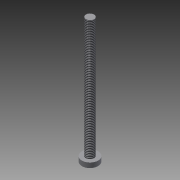
# Autodesk Inventor part: 6-32_Bolt
Saved by Autodesk Inventor 2015 (Build 190159000, 159)
## iProperties
Created: 2017-03-10
Part Number: 6-32_Bolt
Material: Generic
Document SubType Name: Modeling
Designer: Ernest
Density: 1 g/cm^3
Appearance: Default
Author: Ernest
Autodesk Inventor part; units mm, degrees
ref_plane "YZ Plane" through (0, 0, 0) normal (1, 0, 0) x (0, 1, 0)
ref_plane "XZ Plane" through (0, 0, 0) normal (0, 1, 0) x (-1, 0, 0)
ref_plane "XY Plane" through (0, 0, 0) normal (0, 0, 1) x (1, 0, 0)
sketch "Sketch1" plane through (0, 0, 0) normal (0, 0, 1) x (1, 0, 0)
  circle A0 centre (0, 0) radius 3.375
  dimension "d0" = 6.75
  constraints: 1 centre point, 1 coincident
  measures "d0" diameter of A0
extrude "Extrusion1" add sketch "Sketch1" along normal blind 2.6
sketch "Sketch2" plane through (0, 0, 2.6) normal (0, 0, 1) x (1, 0, 0)
  circle A0 centre (0, 0) radius 1.7
  dimension "d3" = 3.4
  constraints: 1 centre point, 1 coincident
  measures "d3" diameter of A0
extrude "Extrusion2" add sketch "Sketch2" along normal blind 50
thread "Thread1" size "M3.5x0.6" class "6g" standard "ANSI Metric M Profile" full length
chamfer "Chamfer1" distance 1.5 angle 20 1 edges at (-3.375, 0, 0) measured on face at (1.1885, -0.5228, 0)
fillet "Fillet1" radius 0.25 2 edges at (-3.375, 0, 0.546) (-1.875, 0, 0)
body "Solid1"
